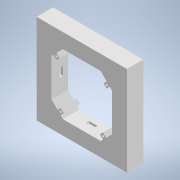
# Autodesk Inventor part: Середина 2
Saved by Autodesk Inventor 2021.2 (Build 252289000, 289)
## iProperties
Created: 2021-11-01
Part Number: Середина 2
Material: Типовые
Document SubType Name: Modeling
Designer: Kolan
Density: 1 g/cm^3
Appearance: По умолчанию
Author: Kolan
Autodesk Inventor part; units mm, degrees
ref_plane "YZ Plane" through (0, 0, 0) normal (1, 0, 0) x (0, 1, 0)
ref_plane "XZ Plane" through (0, 0, 0) normal (0, 1, 0) x (-1, 0, 0)
sketch "Эскиз1" plane through (0, 0, 0) normal (0, 0, 1) x (1, 0, 0)
  circle A0 centre (0, 31.678) radius 1.5 construction
  circle A1 centre (31.678, 0) radius 1.5 construction
  circle A2 centre (-31.678, 0) radius 1.5 construction
  circle A3 centre (0, -31.678) radius 1.5 construction
  line L0 (21.7815, 38.678) -> (-21.7815, 38.678) construction
  line L1 (-21.7815, 38.678) -> (-38.678, 21.7815) construction
  line L2 (-38.678, 21.7815) -> (-38.678, -21.7815) construction
  line L3 (-38.678, -21.7815) -> (-21.7815, -38.678) construction
  line L4 (-21.7815, -38.678) -> (21.7815, -38.678) construction
  line L5 (21.7815, -38.678) -> (38.678, -21.7815) construction
  line L6 (38.678, -21.7815) -> (38.678, 21.7815) construction
  line L7 (38.678, 21.7815) -> (21.7815, 38.678) construction
  line L8 (17.2251, 27.678) -> (22.7283, 22.1749) construction
  line L9 (22.7283, 22.1749) -> (19.8998, 19.3464) construction
  line L10 (19.8998, 19.3464) -> (22.7283, 16.518) construction
  line L11 (22.7283, 16.518) -> (25.5567, 19.3464) construction
  line L12 (25.5567, 19.3464) -> (27.678, 17.2251) construction
  line L13 (27.678, 17.2251) -> (27.678, -17.2251) construction
  line L14 (27.678, -17.2251) -> (22.1749, -22.7283) construction
  line L15 (22.1749, -22.7283) -> (19.3464, -19.8998) construction
  line L16 (19.3464, -19.8998) -> (16.518, -22.7283) construction
  line L17 (16.518, -22.7283) -> (19.3464, -25.5567) construction
  line L18 (19.3464, -25.5567) -> (17.2251, -27.678) construction
  line L19 (17.2251, -27.678) -> (-17.2251, -27.678) construction
  line L20 (-17.2251, -27.678) -> (-19.3464, -25.5567) construction
  line L21 (-19.3464, -25.5567) -> (-16.518, -22.7283) construction
  line L22 (-16.518, -22.7283) -> (-19.3464, -19.8998) construction
  line L23 (-19.3464, -19.8998) -> (-22.1749, -22.7283) construction
  line L24 (-22.1749, -22.7283) -> (-27.678, -17.2251) construction
  line L25 (-27.678, -17.2251) -> (-27.678, 17.2251) construction
  line L26 (-27.678, 17.2251) -> (-25.9871, 18.916) construction
  line L27 (-17.2251, 27.678) -> (17.2251, 27.678) construction
  circle A4 centre (-5, -30.678) radius 1.5 construction
  circle A5 centre (-30.678, 5) radius 1.5 construction
  circle A6 centre (5, 30.678) radius 1.5 construction
  circle A7 centre (30.678, -5) radius 1.5 construction
  line L28 (38.678, 38.678) -> (-38.678, 38.678) construction
  line L29 (-38.678, 38.678) -> (-38.678, -38.178) construction
  line L30 (-38.678, -38.178) -> (38.678, -38.178) construction
  line L31 (38.678, -38.178) -> (38.678, 38.678) construction
  line L32 (-41.178, -40.678) -> (-41.178, 41.178)
  line L33 (-41.178, 41.178) -> (41.178, 41.178)
  line L34 (41.178, 41.178) -> (41.178, -40.678)
  line L35 (41.178, -40.678) -> (-41.178, -40.678)
  line L36 (-39.178, 39.178) -> (-39.178, -38.678)
  line L37 (-39.178, -38.678) -> (39.178, -38.678)
  line L38 (39.178, -38.678) -> (39.178, 39.178)
  line L39 (39.178, 39.178) -> (-39.178, 39.178)
  circle A8 centre (22.7283, 19.3419) radius 1 projected
  circle A9 centre (-19.3738, -22.7283) radius 1 projected
  circle A10 centre (19.3407, -22.734) radius 1 projected
  circle A11 centre (-23.1587, 18.9654) radius 1 projected
  line L40 (-25.9871, 18.916) -> (-23.1587, 16.0876) projected
  line L41 (-23.1587, 16.0876) -> (-20.3302, 18.916) projected
  line L42 (-20.3302, 18.916) -> (-23.1587, 21.7444) projected
  line L43 (-23.1587, 21.7444) -> (-17.2251, 27.678) projected
  point P0 (0, 0)
  dimension "d0" = 2.5
  dimension "d1" = 2
  constraints: 24 end point, 6 parallel, 3 perpendicular, 2 point on line, 1 horizontal, 6 other
  measures "d0" distance between parallel lines of L29 L32
  measures "d1" distance between parallel lines of L32 L36
extrude "Выдавливание1" add sketch "Эскиз1" along normal blind 13 contours L32 L33 L34 L35
sketch "Эскиз2" plane through (0, 0, 13) normal (0, 0, 1) x (1, 0, 0)
  line L0 (41.178, -40.678) -> (-41.178, -40.678)
  line L1 (-41.178, -40.678) -> (-41.178, 41.178)
  line L2 (-41.178, 41.178) -> (41.178, 41.178)
  line L3 (41.178, 41.178) -> (41.178, -40.678)
  circle A0 centre (0, 31.678) radius 1.5 construction
  circle A1 centre (31.678, 0) radius 1.5 construction
  circle A2 centre (-31.678, 0) radius 1.5 construction
  circle A3 centre (0, -31.678) radius 1.5 construction
  line L4 (21.7815, 38.678) -> (-21.7815, 38.678) construction
  line L5 (-21.7815, 38.678) -> (-38.678, 21.7815) construction
  line L6 (-38.678, 21.7815) -> (-38.678, -21.7815) construction
  line L7 (-38.678, -21.7815) -> (-21.7815, -38.678) construction
  line L8 (-21.7815, -38.678) -> (21.7815, -38.678) construction
  line L9 (21.7815, -38.678) -> (38.678, -21.7815) construction
  line L10 (38.678, -21.7815) -> (38.678, 21.7815) construction
  line L11 (38.678, 21.7815) -> (21.7815, 38.678) construction
  line L12 (17.2251, 27.678) -> (22.7283, 22.1749) construction
  line L13 (22.7283, 22.1749) -> (19.8998, 19.3464) construction
  line L14 (19.8998, 19.3464) -> (22.7283, 16.518) construction
  line L15 (22.7283, 16.518) -> (25.5567, 19.3464) construction
  line L16 (25.5567, 19.3464) -> (27.678, 17.2251) construction
  line L17 (27.678, 17.2251) -> (27.678, -17.2251) construction
  line L18 (27.678, -17.2251) -> (22.1749, -22.7283) construction
  line L19 (22.1749, -22.7283) -> (19.3464, -19.8998) construction
  line L20 (19.3464, -19.8998) -> (16.518, -22.7283) construction
  line L21 (16.518, -22.7283) -> (19.3464, -25.5567) construction
  line L22 (19.3464, -25.5567) -> (17.2251, -27.678) construction
  line L23 (17.2251, -27.678) -> (-17.2251, -27.678) construction
  line L24 (-17.2251, -27.678) -> (-19.3464, -25.5567) construction
  line L25 (-19.3464, -25.5567) -> (-16.518, -22.7283) construction
  line L26 (-16.518, -22.7283) -> (-19.3464, -19.8998) construction
  line L27 (-19.3464, -19.8998) -> (-22.1749, -22.7283) construction
  line L28 (-22.1749, -22.7283) -> (-27.678, -17.2251) construction
  line L29 (-27.678, -17.2251) -> (-27.678, 17.2251) construction
  line L30 (-27.678, 17.2251) -> (-17.2251, 27.678) construction
  line L31 (-17.2251, 27.678) -> (17.2251, 27.678) construction
  circle A4 centre (-5, -30.678) radius 1.5 construction
  circle A5 centre (-30.678, 5) radius 1.5 construction
  circle A6 centre (5, 30.678) radius 1.5 construction
  circle A7 centre (30.678, -5) radius 1.5 construction
  circle A8 centre (0, 31.678) radius 1.5 construction
  circle A9 centre (31.678, 0) radius 1.5 construction
  circle A10 centre (-31.678, 0) radius 1.5 construction
  circle A11 centre (0, -31.678) radius 1.5 construction
  line L32 (21.7815, 38.678) -> (-21.7815, 38.678) construction
  line L33 (-21.7815, 38.678) -> (-38.678, 21.7815) construction
  line L34 (-38.678, 21.7815) -> (-38.678, -21.7815) construction
  line L35 (-38.678, -21.7815) -> (-21.7815, -38.678) construction
  line L36 (-21.7815, -38.678) -> (21.7815, -38.678) construction
  line L37 (21.7815, -38.678) -> (38.678, -21.7815) construction
  line L38 (38.678, -21.7815) -> (38.678, 21.7815) construction
  line L39 (38.678, 21.7815) -> (21.7815, 38.678) construction
  line L40 (17.2251, 27.678) -> (22.7283, 22.1749)
  line L41 (22.7283, 22.1749) -> (19.8998, 19.3464)
  line L42 (19.8998, 19.3464) -> (22.7283, 16.518)
  line L43 (22.7283, 16.518) -> (25.5567, 19.3464)
  line L44 (25.5567, 19.3464) -> (27.678, 17.2251)
  line L45 (27.678, 17.2251) -> (27.678, -17.2251)
  line L46 (27.678, -17.2251) -> (22.1749, -22.7283)
  line L47 (22.1749, -22.7283) -> (19.3464, -19.8998)
  line L48 (19.3464, -19.8998) -> (16.518, -22.7283)
  line L49 (16.518, -22.7283) -> (19.3464, -25.5567)
  line L50 (19.3464, -25.5567) -> (17.2251, -27.678)
  line L51 (17.2251, -27.678) -> (-17.2251, -27.678)
  line L52 (-17.2251, -27.678) -> (-19.3464, -25.5567)
  line L53 (-19.3464, -25.5567) -> (-16.518, -22.7283)
  line L54 (-16.518, -22.7283) -> (-19.3464, -19.8998)
  line L55 (-19.3464, -19.8998) -> (-22.1749, -22.7283)
  line L56 (-22.1749, -22.7283) -> (-27.678, -17.2251)
  line L57 (-27.678, -17.2251) -> (-27.678, 17.2251)
  line L58 (-27.678, 17.2251) -> (-17.2251, 27.678)
  line L59 (-17.2251, 27.678) -> (17.2251, 27.678)
  circle A12 centre (-5, -30.678) radius 1.5 construction
  circle A13 centre (-30.678, 5) radius 1.5 construction
  circle A14 centre (5, 30.678) radius 1.5 construction
  circle A15 centre (30.678, -5) radius 1.5 construction
  circle A16 centre (19.3464, -22.7283) radius 1
  circle A17 centre (22.7283, 19.3464) radius 1
  line L60 (-25.9871, 18.916) -> (-23.1587, 16.0876)
  line L61 (-23.1587, 16.0876) -> (-20.3302, 18.916)
  line L62 (-20.3302, 18.916) -> (-23.1587, 21.7444)
  circle A18 centre (-23.1587, 18.9654) radius 1
  circle A19 centre (-19.3738, -22.7283) radius 1
  point P0 (0, 0)
extrude "Выдавливание2" add sketch "Эскиз2" along normal blind 2 contours L0 L1 L2 L3 | L62 L61 L60 L58
sketch "Эскиз3" plane through (0, 0, 13) normal (0, 0, -1) x (-1, 0, 0)
  circle A0 centre (0, 31.678) radius 1.5 construction
  circle A1 centre (-31.678, 0) radius 1.5 construction
  circle A2 centre (31.678, 0) radius 1.5 construction
  circle A3 centre (0, -31.678) radius 1.5 construction
  line L0 (-21.7815, 38.678) -> (21.7815, 38.678) construction
  line L1 (-38.678, 21.7815) -> (-21.7815, 38.678) construction
  line L2 (-38.678, -21.7815) -> (-38.678, 21.7815) construction
  line L3 (-21.7815, -38.678) -> (-38.678, -21.7815) construction
  line L4 (21.7815, -38.678) -> (-21.7815, -38.678) construction
  line L5 (38.678, -21.7815) -> (21.7815, -38.678) construction
  line L6 (38.678, 21.7815) -> (38.678, -21.7815) construction
  line L7 (21.7815, 38.678) -> (38.678, 21.7815) construction
  line L8 (-17.2251, 27.678) -> (-22.7283, 22.1749) construction
  line L9 (17.2251, 27.678) -> (-17.2251, 27.678) construction
  line L10 (27.678, 17.2251) -> (25.9871, 18.916) construction
  line L11 (27.678, -17.2251) -> (27.678, 17.2251) construction
  line L12 (22.1749, -22.7283) -> (27.678, -17.2251) construction
  line L13 (19.3464, -25.5567) -> (22.1749, -22.7283) construction
  line L14 (17.2251, -27.678) -> (19.3464, -25.5567) construction
  line L15 (-17.2251, -27.678) -> (17.2251, -27.678) construction
  line L16 (-19.3464, -25.5567) -> (-17.2251, -27.678) construction
  line L17 (-22.1749, -22.7283) -> (-19.3464, -25.5567) construction
  line L18 (-27.678, -17.2251) -> (-22.1749, -22.7283) construction
  line L19 (-27.678, 17.2251) -> (-27.678, -17.2251) construction
  line L20 (-25.5567, 19.3464) -> (-27.678, 17.2251) construction
  line L21 (-22.7283, 22.1749) -> (-25.5567, 19.3464) construction
  circle A4 centre (5, -30.678) radius 1.5 construction
  circle A5 centre (30.678, 5) radius 1.5 construction
  circle A6 centre (-5, 30.678) radius 1.5 construction
  circle A7 centre (-30.678, -5) radius 1.5 construction
  line L22 (18.0535, -29.678) -> (-18.0535, -29.678)
  line L23 (-18.0535, -29.678) -> (-29.678, -18.0535)
  line L24 (-29.678, -18.0535) -> (-29.678, 18.0535)
  line L25 (-29.678, 18.0535) -> (-18.0535, 29.678)
  line L26 (-18.0535, 29.678) -> (18.0535, 29.678)
  line L27 (18.0535, 29.678) -> (29.678, 18.0535)
  line L28 (29.678, 18.0535) -> (29.678, -18.0535)
  line L29 (29.678, -18.0535) -> (18.0535, -29.678)
  line L30 (17.2251, -27.678) -> (-17.2251, -27.678)
  line L31 (-27.678, -17.2251) -> (-27.678, 17.2251)
  line L32 (-17.2251, 27.678) -> (17.2251, 27.678)
  line L33 (27.678, 17.2251) -> (27.678, -17.2251)
  line L34 (16.518, -22.7283) -> (19.3464, -25.5567) projected
  line L35 (19.3464, -19.8998) -> (16.518, -22.7283) projected
  line L36 (22.1749, -22.7283) -> (19.3464, -19.8998) projected
  line L37 (-25.5567, 19.3464) -> (-22.7283, 16.518) projected
  line L38 (-22.7283, 16.518) -> (-19.8998, 19.3464) projected
  line L39 (-19.8998, 19.3464) -> (-22.7283, 22.1749) projected
  circle A8 centre (-22.7283, 19.3464) radius 1 projected
  line L40 (-19.3464, -25.5567) -> (-16.518, -22.7283) projected
  line L41 (-16.518, -22.7283) -> (-19.3464, -19.8998) projected
  line L42 (-19.3464, -19.8998) -> (-22.1749, -22.7283) projected
  circle A9 centre (-19.3464, -22.7283) radius 1 projected
  line L43 (27.678, -17.2251) -> (22.1749, -22.7283)
  line L44 (19.3464, -25.5567) -> (17.2251, -27.678)
  line L45 (-27.678, 17.2251) -> (-25.5567, 19.3464)
  line L46 (-22.7283, 22.1749) -> (-17.2251, 27.678)
  line L47 (-17.2251, -27.678) -> (-19.3464, -25.5567)
  line L48 (-22.1749, -22.7283) -> (-27.678, -17.2251)
  line L49 (23.1587, 21.7444) -> (17.2251, 27.678) projected
  line L50 (25.9871, 18.916) -> (23.1587, 21.7444) projected
  circle A10 centre (19.3738, -22.7283) radius 1 projected
  circle A11 centre (23.1587, 18.9654) radius 1 projected
  line L51 (20.3302, 18.916) -> (23.1587, 21.7444) projected
  line L52 (23.1587, 16.0876) -> (20.3302, 18.916) projected
  line L53 (25.9871, 18.916) -> (23.1587, 16.0876) projected
  line L54 (17.2251, 27.678) -> (23.1587, 21.7444)
  line L55 (25.9871, 18.916) -> (27.678, 17.2251)
  point P0 (0, 0)
  dimension "d9" = 9
  constraints: 44 end point, 4 point on line, 7 other
  measures "d9" distance between parallel lines of L5 L29
ref_plane "РабПлоскость1" through (-38.678, -38.678, 0) normal (0, 0, 1) x (1, 0, 0)
extrude "Выдавливание3" add sketch "Эскиз3" along normal up to surface (13 mm away) contours L22 L23 L24 L25 L26 L27 L28 L29 | L53 L52 L51 L50
sketch "Эскиз4" plane through (-27.678, -17.2251, 15) normal (1, 0, 0) x (0, 0, -1)
  line L0 (10, 20.2251) -> (10, 14.2251) construction
  line L1 (10.5, 20.2251) -> (10.5, 14.2251)
  line L2 (7.5, 20.2251) -> (7.5, 14.2251)
  line L3 (15, 58.4031) -> (15, -23.4529) projected
  line L4 (7.5, 20.2251) -> (7.5, 20.9751)
  line L5 (7.5, 20.9751) -> (10.5, 20.9751)
  line L6 (10.5, 20.9751) -> (10.5, 20.2251)
  line L7 (7.5, 14.2251) -> (7.5, 13.4751)
  line L8 (7.5, 13.4751) -> (10.5, 13.4751)
  line L9 (10.5, 13.4751) -> (10.5, 14.2251)
  point P0 (15, 17.2251)
  dimension "d13" = 0.5
  dimension "d14" = 2.5
  dimension "d18" = 0.75
  dimension "d19" = 0.75
  constraints: 16 end point, 4 perpendicular, 2 parallel, 2 vertical
  measures "d13" distance between parallel lines of L0 L1
  measures "d14" distance between parallel lines of L0 L2
  measures "d18" distance of L2.start L4.end
  measures "d19" distance of L2.end L7.end
extrude "Выдавливание4" cut sketch "Эскиз4" against normal up to surface (2 mm away)
sketch "Эскиз5" plane through (-17.2251, 27.678, 15) normal (0, -1, 0) x (1, 0, 0)
  line L0 (20.2251, -10) -> (14.2251, -10) construction
  line L1 (20.2251, -10.5) -> (14.2251, -10.5)
  line L2 (20.2251, -7.5) -> (14.2251, -7.5)
  line L3 (20.2251, -7.5) -> (20.9751, -7.5)
  line L4 (20.9751, -7.5) -> (20.9751, -10.5)
  line L5 (20.9751, -10.5) -> (20.2251, -10.5)
  line L6 (14.2251, -7.5) -> (13.4751, -7.5)
  line L7 (13.4751, -7.5) -> (13.4751, -10.5)
  line L8 (13.4751, -10.5) -> (14.2251, -10.5)
  point P0 (17.2251, -15)
  dimension "d20" = 0.5
  dimension "d21" = 2.5
  dimension "d22" = 0.75
  dimension "d23" = 0.75
  constraints: 16 end point, 3 perpendicular, 2 horizontal, 2 parallel, 1 vertical
  measures "d20" distance between parallel lines of L0 L1
  measures "d21" distance between parallel lines of L0 L2
  measures "d22" distance of L2.start L3.end
  measures "d23" distance of L2.end L6.end
extrude "Выдавливание5" cut sketch "Эскиз5" against normal up to surface (2 mm away)
sketch "Эскиз6" plane through (27.678, -17.2251, 15) normal (-1, 0, 0) x (0, 0, 1)
  line L0 (-10, 14.2251) -> (-10, 20.2251) construction
  line L1 (-10.5, 14.2251) -> (-10.5, 20.2251)
  line L2 (-7.5, 14.2251) -> (-7.5, 20.2251)
  line L3 (-7.5, 14.2251) -> (-7.5, 13.4751)
  line L4 (-7.5, 13.4751) -> (-10.5, 13.4751)
  line L5 (-10.5, 13.4751) -> (-10.5, 14.2251)
  line L6 (-7.5, 20.2251) -> (-7.5, 20.9751)
  line L7 (-7.5, 20.9751) -> (-10.5, 20.9751)
  line L8 (-10.5, 20.9751) -> (-10.5, 20.2251)
  point P0 (-15, 17.2251)
  dimension "d26" = 0.5
  dimension "d27" = 2.5
  dimension "d28" = 0.75
  dimension "d29" = 0.75
  constraints: 16 end point, 4 perpendicular, 2 parallel, 2 vertical
  measures "d26" distance between parallel lines of L0 L1
  measures "d27" distance between parallel lines of L0 L2
  measures "d28" distance of L2.start L3.end
  measures "d29" distance of L2.end L6.end
extrude "Выдавливание6" cut sketch "Эскиз6" against normal up to surface (2 mm away)
sketch "Эскиз7" plane through (-17.2251, -27.678, 15) normal (0, 1, 0) x (1, 0, 0)
  line L0 (14.2251, 10) -> (20.2251, 10) construction
  line L1 (14.2251, 10.5) -> (20.2251, 10.5)
  line L2 (14.2251, 7.5) -> (20.2251, 7.5)
  line L3 (20.2251, 7.5) -> (20.9751, 7.5)
  line L4 (56.4031, 15) -> (-21.9529, 15) projected
  line L5 (20.9751, 7.5) -> (20.9751, 10.5)
  line L6 (20.9751, 10.5) -> (20.2251, 10.5)
  line L7 (14.2251, 7.5) -> (13.4751, 7.5)
  line L8 (13.4751, 7.5) -> (13.4751, 10.5)
  line L9 (13.4751, 10.5) -> (14.2251, 10.5)
  point P0 (17.2251, 15)
  dimension "d32" = 0.5
  dimension "d33" = 2.5
  dimension "d34" = 0.75
  dimension "d35" = 0.75
  constraints: 16 end point, 4 perpendicular, 3 parallel, 2 point on line
  measures "d32" distance between parallel lines of L0 L1
  measures "d33" distance between parallel lines of L0 L2
  measures "d34" distance of L2.end L3.end
  measures "d35" distance of L2.start L7.end
extrude "Выдавливание7" cut sketch "Эскиз7" against normal up to surface (2 mm away)
